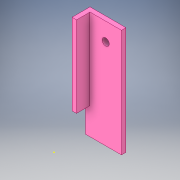
# Autodesk Inventor part: LiftAngleBracketExtensionLeft
Saved by Autodesk Inventor 2017 SP1 (Build 210196100, 196)
## iProperties
Created: 2016-08-26
Part Number: LiftAngleBracketExtensionLeft
Material: Aluminum 6061
Document SubType Name: Modeling
Designer: steele
Density: 2.7 g/cm^3
Appearance: Pink
Author: steele
Autodesk Inventor part; units mm, degrees
ref_plane "YZ Plane" through (0, 0, 0) normal (1, 0, 0) x (0, 1, 0)
ref_plane "XZ Plane" through (0, 0, 0) normal (0, 1, 0) x (-1, 0, 0)
ref_plane "XY Plane" through (0, 0, 0) normal (0, 0, 1) x (1, 0, 0)
sketch "Sketch1" plane through (0, 0, 0) normal (0, 1, 0) x (-1, 0, 0)
  line L0 (0, 0) -> (0, -50.8)
  line L1 (0, -50.8) -> (-50.8, -50.8)
  line L2 (-50.8, -50.8) -> (-50.8, -44.45)
  line L3 (-50.8, -44.45) -> (-6.35, -44.45)
  line L4 (-6.35, -44.45) -> (-6.35, 0)
  line L5 (-6.35, 0) -> (0, 0)
  dimension "d0" = 6.35
  dimension "d1" = 50.8
  constraints: 12 end point, 7 perpendicular, 1 vertical
  measures "d0" distance of L4.end L0.start
  measures "d1" distance of L0.end L1.end
extrude "Extrusion1" add sketch "Sketch1" along normal blind 152.4
sketch "Sketch2" plane through (0, 0, -50.8) normal (-1, 0, 0) x (0, 0, 1)
  point P0 (50.8, 0)
sketch "Sketch3" plane through (6.35, 0, 0) normal (1, 0, 0) x (0, 0, -1)
  line L0 (0, 0) -> (50.8, 0) projected
  line L1 (44.45, 0) -> (44.45, 152.4) projected
  line L2 (0, 0) -> (44.45, 0)
  line L3 (44.45, 0) -> (44.45, 38.1)
  line L4 (44.45, 38.1) -> (0, 38.1)
  line L5 (0, 38.1) -> (0, 0)
  dimension "d5" = 38.1
  constraints: 8 end point, 2 parallel, 1 horizontal, 1 perpendicular, 1 point on line
  measures "d5" distance of L4.end L0.start
extrude "Extrusion2" cut sketch "Sketch3" against normal through all
sketch "Sketch4" plane through (6.35, 152.4, 0) normal (1, 0, 0) x (0, 0, -1)
  line L0 (0, -114.3) -> (0, 0) projected
  line L1 (50.8, 0) -> (0, 0) projected
  line L2 (0, -114.3) -> (25.4, -114.3)
  line L3 (25.4, -114.3) -> (25.4, 0)
  line L4 (25.4, 0) -> (0, 0)
  line L5 (0, 0) -> (0, -114.3)
  point P0 (0, -152.4)
  dimension "d8" = 25.4
  constraints: 8 end point, 2 parallel, 1 horizontal, 1 midpoint, 1 perpendicular
  measures "d8" distance between parallel lines of L3 L0
extrude "Extrusion3" cut sketch "Sketch4" against normal through all
sketch "Sketch6" plane through (50.8, 0, -50.8) normal (0, 0, -1) x (-1, 0, 0)
  line L0 (0, 152.4) -> (50.8, 152.4) projected
  line L1 (0, 0) -> (0, 152.4) projected
  point P0 (50.8, 0)
  point P1 (22.225, 127)
  dimension "d11" = 25.4
  dimension "d12" = 22.225
  measures "d11" distance from line of point (22.225, 127) L0
  measures "d12" distance from line of point (22.225, 127) L1
hole "Hole1" at (28.575, 127, -50.8) direction (0, 0, 1) diameter 10.0838 end through all clearance for "Flat Head Machine Screw (82)" size "3/8" standard "Ansi Unified Screw Threads"
body "Solid1"
